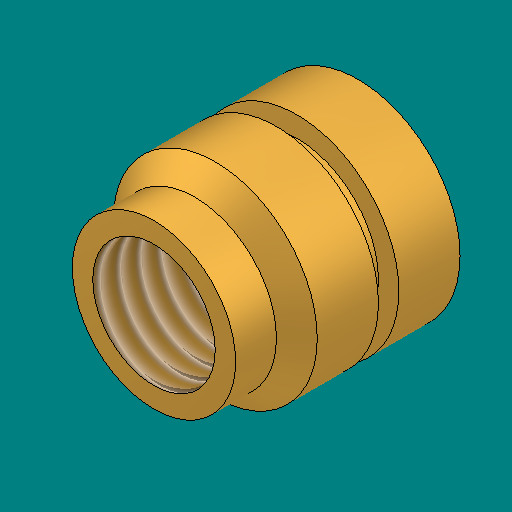
# Autodesk Inventor part: brass-insert-m3x5
Saved by Autodesk Inventor 2025 (Build 290162000, 162)
## iProperties
Created: 2024-07-09
Part Number: brass-insert-m3x5
Material: Brass, Soft Yellow
Document SubType Name: Modeling
Designer: kuzmin
Density: 8.47 g/cm^3
Appearance: Brass - Satin
Author: kuzmin
Autodesk Inventor part; units mm, degrees
ref_plane "YZ Plane" through (0, 0, 0) normal (1, 0, 0) x (0, 1, 0)
ref_plane "XZ Plane" through (0, 0, 0) normal (0, 1, 0) x (-1, 0, 0)
ref_plane "XY Plane" through (0, 0, 0) normal (0, 0, 1) x (1, 0, 0)
sketch "Sketch1" plane through (0, 0, 0) normal (0, 1, 0) x (-1, 0, 0)
  line L0 (0, 0) -> (0, 5)
  line L1 (0, 5) -> (2, 5)
  line L2 (2, 5) -> (2, 3.5)
  line L3 (2, 3.5) -> (2.5, 3.5)
  line L4 (2.5, 3.5) -> (2.5, 2)
  line L5 (2.5, 2) -> (2, 2)
  line L6 (2, 2) -> (2, 1.5)
  line L7 (2, 1.5) -> (2.5, 1.5)
  line L8 (2.5, 1.5) -> (2.5, 0)
  line L9 (2.5, 0) -> (0, 0)
  dimension "d0" = 5
  dimension "d1" = 5
  dimension "d2" = 4
  dimension "d3" = 1.5
  dimension "d4" = 0.5
  dimension "d5" = 1.5
  constraints: 20 end point, 6 perpendicular, 4 point on line, 1 horizontal, 1 vertical
  measures "d0" distance between parallel lines of L9 L1
  measures "d1" diameter of L8 L0
  measures "d2" diameter of L2 L0
  measures "d3" distance of L7.end L8.end
  measures "d4" distance of L5.end L6.end
  measures "d5" distance of L3.end L4.end
revolve "Revolution1" add sketch "Sketch1" angle 360 about axis through (0, 0, 0) along (0, 0, 1)
chamfer "Chamfer1" distance 0.5 angle 45 1 edges at (2, 0, 3.5)
hole "Hole1" at (0, 0, 0) direction (0, 0, 1) diameter 3 depth 6 tip angle 118
thread "Thread1" size "M3x0.5" class "6H" standard "ANSI Metric M Profile" full length
body "Solid1"
